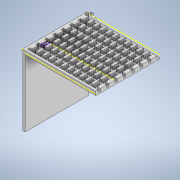
# Autodesk Inventor part: Garbage collectorBar
Saved by Autodesk Inventor 2022 (Build 260153000, 153)
## iProperties
Created: 2022-03-28
Part Number: Garbage collectorBar
Material: Generic
Document SubType Name: Modeling
Designer: Aditya Gupte
Density: 1 g/cm^3
Appearance: Default
Author: Aditya Gupte
Autodesk Inventor part; units mm, degrees
ref_plane "YZ Plane" through (0, 0, 0) normal (1, 0, 0) x (0, 1, 0)
ref_plane "XZ Plane" through (0, 0, 0) normal (0, 1, 0) x (-1, 0, 0)
ref_plane "XY Plane" through (0, 0, 0) normal (0, 0, 1) x (1, 0, 0)
sketch "Sketch1" plane through (0, 0, 0) normal (0, 0, 1) x (1, 0, 0)
  line L0 (0, 0) -> (15000, 0)
  line L1 (0, 0) -> (0, 14450)
  line L2 (0, 14450) -> (500, 14450)
  line L3 (500, 14450) -> (500, 300)
  line L4 (500, 300) -> (14950, 300)
  line L5 (14950, 300) -> (14950, 0)
  dimension "d0" = 15000
  dimension "d1" = 14450
  dimension "d2" = 500
  dimension "d3" = 14150
  dimension "d4" = 14450
  constraints: 12 end point, 3 perpendicular, 2 horizontal, 1 point on line, 1 vertical
  measures "d0" distance of L0.start L0.end
  measures "d1" distance of L0.start L1.end
  measures "d2" distance of L1.end L2.end
  measures "d3" distance of L2.end L3.end
  measures "d4" distance of L3.end L4.end
extrude "Extrusion1" add sketch "Sketch1" against normal blind 13000
sketch "Sketch2" plane through (500, 300, 0) normal (0, 1, 0) x (1, 0, 0)
  line L0 (14450, 0) -> (0, 0) projected
  line L1 (0, 0) -> (0, 13000) projected
  line L2 (-500, 0) -> (-500, 13000) projected
  dimension "d8" = 500
  measures "d8" distance between parallel lines of L1 L2
sketch "Sketch3" plane through (500, 300, 0) normal (0, 1, 0) x (1, 0, 0)
  line L0 (14450, 0) -> (14450, 13000) projected
  line L1 (14450, 0) -> (0, 0) projected
  line L2 (14450, 450) -> (0, 450)
  line L3 (14450, 950) -> (0, 950)
  line L4 (0, 0) -> (0, 13000) projected
  line L5 (0, 0) -> (0, 450)
  line L6 (14450, 0) -> (14450, 450)
  line L7 (0, 950) -> (14450, 950)
  line L8 (14450, 950) -> (14450, 2170)
  line L9 (14450, 2170) -> (0, 2170)
  line L10 (0, 2170) -> (0, 950)
  line L11 (0, 2670) -> (14450, 2670)
  line L12 (14450, 2670) -> (14450, 3890)
  line L13 (14450, 3890) -> (0, 3890)
  line L14 (0, 3890) -> (0, 2670)
  line L15 (0, 4390) -> (14450, 4390)
  line L16 (14450, 4390) -> (14450, 5610)
  line L17 (14450, 5610) -> (0, 5610)
  line L18 (0, 5610) -> (0, 4390)
  line L19 (0, 6110) -> (14450, 6110)
  line L20 (14450, 6110) -> (14450, 7330)
  line L21 (14450, 7330) -> (0, 7330)
  line L22 (0, 7330) -> (0, 6110)
  line L23 (0, 7830) -> (14450, 7830)
  line L24 (14450, 7830) -> (14450, 9050)
  line L25 (14450, 9050) -> (0, 9050)
  line L26 (0, 9050) -> (0, 7830)
  line L27 (0, 9550) -> (14450, 9550)
  line L28 (14450, 9550) -> (14450, 10770)
  line L29 (14450, 10770) -> (0, 10770)
  line L30 (0, 10770) -> (0, 9550)
  line L31 (0, 11270) -> (14450, 11270)
  line L32 (14450, 11270) -> (14450, 12490)
  line L33 (14450, 12490) -> (0, 12490)
  line L34 (0, 12490) -> (0, 11270)
  point P0 (-500, 0)
  point P1 (0, 5610)
  point P2 (0, 7330)
  point P3 (0, 10770)
  point P4 (0, 12490)
  dimension "d9" = 450
  dimension "d10" = 14450
  dimension "d11" = 14450
  dimension "d12" = 500
  dimension "d13" = 1220
  dimension "d14" = 500
  dimension "d15" = 1220
  dimension "d16" = 1220
  dimension "d17" = 500
  dimension "d18" = 1220
  dimension "d19" = 500
  dimension "d20" = 1220
  dimension "d21" = 500
  dimension "d22" = 1220
  dimension "d23" = 500
  dimension "d24" = 1220
  dimension "d25" = 500
  constraints: 64 end point, 14 parallel, 9 horizontal, 7 perpendicular, 1 vertical, 17 other
  measures "d9" distance from line of L2.start L1
  measures "d10" distance of L2.start L2.end
  measures "d11" distance of L3.start L3.end
  measures "d12" distance between parallel lines of L3 L2
  measures "d13" distance of L8.end L7.end
  measures "d14" distance between parallel lines of L11 L9
  measures "d15" distance of L11.end L12.end
  measures "d16" distance of L16.end L15.end
  measures "d17" distance between parallel lines of L15 L13
  measures "d18" distance of L20.end L19.end
  measures "d19" distance between parallel lines of L19 L17
  measures "d20" distance of L24.end L23.end
  measures "d21" distance between parallel lines of L23 L21
  measures "d22" distance of L28.end L27.end
  measures "d23" distance between parallel lines of L27 L25
  measures "d24" distance of L32.end L31.end
  measures "d25" distance between parallel lines of L31 L29
extrude "Extrusion2" add sketch "Sketch3" along normal blind 500 contours L3 L4 L9 L0 | L11 L4 L13 L0 | L15 L4 L17 L0 | L19 L4 L21 L0 | L23 L4 L25 L0 | L27 L4 L29 L0 | L31 L4 L33 L0
sketch "Sketch4" plane through (500, 300, 0) normal (0, 1, 0) x (1, 0, 0)
  line L0 (0, 0) -> (0, 13000) projected
  line L1 (14450, 0) -> (14450, 13000) projected
  line L2 (0, 0) -> (14450, 0)
  line L3 (14450, 0) -> (14450, 450)
  line L4 (14450, 450) -> (0, 450)
  line L5 (0, 450) -> (0, 0)
  point P0 (-500, 0)
  dimension "d28" = 450
  constraints: 8 end point, 2 parallel, 1 horizontal, 1 perpendicular, 1 point on line
  measures "d28" distance of L3.end L2.end
extrude "Extrusion3" add sketch "Sketch4" along normal blind 500
sketch "Sketch5" plane through (500, 800, 0) normal (0, 1, 0) x (1, 0, 0)
  line L0 (0, 12490) -> (14450, 12490) projected
  line L1 (0, 11270) -> (14450, 11270) projected
  line L2 (500, 12490) -> (1250, 12490)
  line L3 (1250, 12490) -> (1250, 11270)
  line L4 (1250, 11270) -> (500, 11270)
  line L5 (500, 11270) -> (500, 12490)
  line L6 (0, 0) -> (0, 13000) projected
  line L7 (1750, 12490) -> (2500, 12490)
  line L8 (2500, 12490) -> (2500, 11270)
  line L9 (2500, 11270) -> (1750, 11270)
  line L10 (1750, 11270) -> (1750, 12490)
  line L11 (3000, 12490) -> (3750, 12490)
  line L12 (3750, 12490) -> (3750, 11270)
  line L13 (3750, 11270) -> (3000, 11270)
  line L14 (3000, 11270) -> (3000, 12490)
  line L15 (4250, 12490) -> (5000, 12490)
  line L16 (5000, 12490) -> (5000, 11270)
  line L17 (5000, 11270) -> (4250, 11270)
  line L18 (4250, 11270) -> (4250, 12490)
  line L19 (5500, 12490) -> (6250, 12490)
  line L20 (6250, 12490) -> (6250, 11270)
  line L21 (6250, 11270) -> (5500, 11270)
  line L22 (5500, 11270) -> (5500, 12490)
  line L23 (6750, 12490) -> (7500, 12490)
  line L24 (7500, 12490) -> (7500, 11270)
  line L25 (7500, 11270) -> (6750, 11270)
  line L26 (6750, 11270) -> (6750, 12490)
  line L27 (8000, 12490) -> (8750, 12490)
  line L28 (8750, 12490) -> (8750, 11270)
  line L29 (8750, 11270) -> (8000, 11270)
  line L30 (8000, 11270) -> (8000, 12490)
  line L31 (9250, 12490) -> (10000, 12490)
  line L32 (10000, 12490) -> (10000, 11270)
  line L33 (10000, 11270) -> (9250, 11270)
  line L34 (9250, 11270) -> (9250, 12490)
  line L35 (10500, 12490) -> (11250, 12490)
  line L36 (11250, 12490) -> (11250, 11270)
  line L37 (11250, 11270) -> (10500, 11270)
  line L38 (10500, 11270) -> (10500, 12490)
  line L39 (11750, 12490) -> (12500, 12490)
  line L40 (12500, 12490) -> (12500, 11270)
  line L41 (12500, 11270) -> (11750, 11270)
  line L42 (11750, 11270) -> (11750, 12490)
  line L43 (13000, 12490) -> (13750, 12490)
  line L44 (13750, 12490) -> (13750, 11270)
  line L45 (13750, 11270) -> (13000, 11270)
  line L46 (13000, 11270) -> (13000, 12490)
  point P0 (-500, 0)
  point P1 (2500, 12490)
  point P2 (500, 11270)
  point P3 (1250, 12490)
  dimension "d31" = 750
  dimension "d32" = 500
  dimension "d33" = 750
  dimension "d34" = 500
  dimension "d35" = 750
  dimension "d36" = 500
  dimension "d37" = 750
  dimension "d38" = 500
  dimension "d39" = 750
  dimension "d40" = 500
  dimension "d41" = 750
  dimension "d42" = 500
  dimension "d43" = 750
  dimension "d44" = 500
  dimension "d45" = 750
  dimension "d46" = 500
  dimension "d47" = 750
  dimension "d48" = 500
  dimension "d49" = 750
  dimension "d50" = 500
  dimension "d51" = 750
  dimension "d52" = 500
  constraints: 88 end point, 22 parallel, 11 horizontal, 11 perpendicular, 24 other
  measures "d31" distance of L3.end L4.end
  measures "d32" distance between parallel lines of L5 L6
  measures "d33" distance of L8.end L9.end
  measures "d34" distance between parallel lines of L10 L3
  measures "d35" distance of L12.end L13.end
  measures "d36" distance between parallel lines of L14 L8
  measures "d37" distance of L16.end L17.end
  measures "d38" distance between parallel lines of L18 L12
  measures "d39" distance of L20.end L21.end
  measures "d40" distance between parallel lines of L22 L16
  measures "d41" distance of L24.end L25.end
  measures "d42" distance between parallel lines of L26 L20
  measures "d43" distance of L28.end L29.end
  measures "d44" distance between parallel lines of L30 L24
  measures "d45" distance of L32.end L33.end
  measures "d46" distance between parallel lines of L34 L28
  measures "d47" distance of L36.end L37.end
  measures "d48" distance between parallel lines of L38 L32
  measures "d49" distance of L40.end L41.end
  measures "d50" distance between parallel lines of L42 L36
  measures "d51" distance of L44.end L45.end
  measures "d52" distance between parallel lines of L46 L40
extrude "Extrusion4" cut sketch "Sketch5" against normal through all contours L0 L3 L1 L5 | L0 L8 L1 L10 | L0 L12 L1 L14 | L0 L16 L1 L18 | L0 L20 L1 L22 | L0 L24 L1 L26 | L0 L28 L1 L30 | L0 L32 L1 L34 | L0 L36 L1 L38 | L0 L40 L1 L42 | L0 L44 L1 L46
sketch "Sketch6" plane through (500, 800, 0) normal (0, 1, 0) x (1, 0, 0)
  line L0 (14450, 10770) -> (0, 10770) projected
  line L1 (14450, 9550) -> (0, 9550) projected
  line L2 (500, 10770) -> (1250, 10770)
  line L3 (1250, 10770) -> (1250, 9550)
  line L4 (1250, 9550) -> (500, 9550)
  line L5 (500, 9550) -> (500, 10770)
  line L6 (0, 0) -> (0, 13000) projected
  line L7 (1750, 10770) -> (2500, 10770)
  line L8 (2500, 10770) -> (2500, 9550)
  line L9 (2500, 9550) -> (1750, 9550)
  line L10 (1750, 9550) -> (1750, 10770)
  line L11 (3000, 10770) -> (3750, 10770)
  line L12 (3750, 10770) -> (3750, 9550)
  line L13 (3750, 9550) -> (3000, 9550)
  line L14 (3000, 9550) -> (3000, 10770)
  line L15 (4250, 10770) -> (5000, 10770)
  line L16 (5000, 10770) -> (5000, 9550)
  line L17 (5000, 9550) -> (4250, 9550)
  line L18 (4250, 9550) -> (4250, 10770)
  line L19 (5500, 10770) -> (6250, 10770)
  line L20 (6250, 10770) -> (6250, 9550)
  line L21 (6250, 9550) -> (5500, 9550)
  line L22 (5500, 9550) -> (5500, 10770)
  line L23 (6750, 10770) -> (7500, 10770)
  line L24 (7500, 10770) -> (7500, 9550)
  line L25 (7500, 9550) -> (6750, 9550)
  line L26 (6750, 9550) -> (6750, 10770)
  line L27 (8000, 10770) -> (8750, 10770)
  line L28 (8750, 10770) -> (8750, 9550)
  line L29 (8750, 9550) -> (8000, 9550)
  line L30 (8000, 9550) -> (8000, 10770)
  line L31 (9250, 10770) -> (10000, 10770)
  line L32 (10000, 10770) -> (10000, 9550)
  line L33 (10000, 9550) -> (9250, 9550)
  line L34 (9250, 9550) -> (9250, 10770)
  line L35 (10500, 10770) -> (11250, 10770)
  line L36 (11250, 10770) -> (11250, 9550)
  line L37 (11250, 9550) -> (10500, 9550)
  line L38 (10500, 9550) -> (10500, 10770)
  line L39 (11750, 10770) -> (12500, 10770)
  line L40 (12500, 10770) -> (12500, 9550)
  line L41 (12500, 9550) -> (11750, 9550)
  line L42 (11750, 9550) -> (11750, 10770)
  line L43 (13000, 10770) -> (13750, 10770)
  line L44 (13750, 10770) -> (13750, 9550)
  line L45 (13750, 9550) -> (13000, 9550)
  line L46 (13000, 9550) -> (13000, 10770)
  line L47 (0, 9050) -> (14450, 9050) projected
  line L48 (500, 9050) -> (1250, 9050)
  line L49 (1250, 9050) -> (1250, 7803.8278)
  line L50 (1250, 7803.8278) -> (500, 7803.8278)
  line L51 (500, 7803.8278) -> (500, 9050)
  line L52 (1750, 9050) -> (2500, 9050)
  line L53 (2500, 9050) -> (2500, 7803.8278)
  line L54 (2500, 7803.8278) -> (1750, 7803.8278)
  line L55 (1750, 7803.8278) -> (1750, 9050)
  line L56 (3000, 9050) -> (3750, 9050)
  line L57 (3750, 9050) -> (3750, 7803.8278)
  line L58 (3750, 7803.8278) -> (3000, 7803.8278)
  line L59 (3000, 7803.8278) -> (3000, 9050)
  line L60 (4250, 9050) -> (5000, 9050)
  line L61 (5000, 9050) -> (5000, 7803.8278)
  line L62 (5000, 7803.8278) -> (4250, 7803.8278)
  line L63 (4250, 7803.8278) -> (4250, 9050)
  line L64 (5500, 9050) -> (6250, 9050)
  line L65 (6250, 9050) -> (6250, 7803.8278)
  line L66 (6250, 7803.8278) -> (5500, 7803.8278)
  line L67 (5500, 7803.8278) -> (5500, 9050)
  line L68 (6750, 9050) -> (7500, 9050)
  line L69 (7500, 9050) -> (7500, 7803.8278)
  line L70 (7500, 7803.8278) -> (6750, 7803.8278)
  line L71 (6750, 7803.8278) -> (6750, 9050)
  line L72 (8000, 9050) -> (8750, 9050)
  line L73 (8750, 9050) -> (8750, 7803.8278)
  line L74 (8750, 7803.8278) -> (8000, 7803.8278)
  line L75 (8000, 7803.8278) -> (8000, 9050)
  line L76 (0, 7830) -> (14450, 7830) projected
  line L77 (9250, 9050) -> (10000, 9050)
  line L78 (10000, 9050) -> (10000, 7830)
  line L79 (10000, 7830) -> (9250, 7830)
  line L80 (9250, 7830) -> (9250, 9050)
  line L81 (10500, 9050) -> (11250, 9050)
  line L82 (11250, 9050) -> (11250, 7830)
  line L83 (11250, 7830) -> (10500, 7830)
  line L84 (10500, 7830) -> (10500, 9050)
  line L85 (11750, 9050) -> (12500, 9050)
  line L86 (12500, 9050) -> (12500, 7830)
  line L87 (12500, 7830) -> (11750, 7830)
  line L88 (11750, 7830) -> (11750, 9050)
  line L89 (13000, 9050) -> (13750, 9050)
  line L90 (13750, 9050) -> (13750, 7830)
  line L91 (13750, 7830) -> (13000, 7830)
  line L92 (13000, 7830) -> (13000, 9050)
  line L93 (14450, 6110) -> (0, 6110) projected
  line L94 (500, 7312.9157) -> (1250, 7312.9157)
  line L95 (1250, 7312.9157) -> (1250, 6110)
  line L96 (1250, 6110) -> (500, 6110)
  line L97 (500, 6110) -> (500, 7312.9157)
  line L98 (1750, 7312.9157) -> (2500, 7312.9157)
  line L99 (2500, 7312.9157) -> (2500, 6110)
  line L100 (2500, 6110) -> (1750, 6110)
  line L101 (1750, 6110) -> (1750, 7312.9157)
  line L102 (3000, 7312.9157) -> (3750, 7312.9157)
  line L103 (3750, 7312.9157) -> (3750, 6110)
  line L104 (3750, 6110) -> (3000, 6110)
  line L105 (3000, 6110) -> (3000, 7312.9157)
  line L106 (4250, 7312.9157) -> (5000, 7312.9157)
  line L107 (5000, 7312.9157) -> (5000, 6110)
  line L108 (5000, 6110) -> (4250, 6110)
  line L109 (4250, 6110) -> (4250, 7312.9157)
  line L110 (0, 7330) -> (14450, 7330) projected
  line L111 (5500, 7330) -> (6250, 7330)
  line L112 (6250, 7330) -> (6250, 6110)
  line L113 (6250, 6110) -> (5500, 6110)
  line L114 (5500, 6110) -> (5500, 7330)
  line L115 (6750, 7330) -> (7500, 7330)
  line L116 (7500, 7330) -> (7500, 6110)
  line L117 (7500, 6110) -> (6750, 6110)
  line L118 (6750, 6110) -> (6750, 7330)
  line L119 (8000, 7330) -> (8750, 7330)
  line L120 (8750, 7330) -> (8750, 6110)
  line L121 (8750, 6110) -> (8000, 6110)
  line L122 (8000, 6110) -> (8000, 7330)
  line L123 (9250, 7330) -> (10000, 7330)
  line L124 (10000, 7330) -> (10000, 6110)
  line L125 (10000, 6110) -> (9250, 6110)
  line L126 (9250, 6110) -> (9250, 7330)
  line L127 (10500, 7330) -> (11250, 7330)
  line L128 (11250, 7330) -> (11250, 6110)
  line L129 (11250, 6110) -> (10500, 6110)
  line L130 (10500, 6110) -> (10500, 7330)
  line L131 (11750, 7330) -> (12500, 7330)
  line L132 (12500, 7330) -> (12500, 6110)
  line L133 (12500, 6110) -> (11750, 6110)
  line L134 (11750, 6110) -> (11750, 7330)
  line L135 (13000, 7312.9157) -> (13750, 7312.9157)
  line L136 (13750, 7312.9157) -> (13750, 6110)
  line L137 (13750, 6110) -> (13000, 6110)
  line L138 (13000, 6110) -> (13000, 7312.9157)
  line L139 (14450, 4390) -> (0, 4390) projected
  line L140 (500, 5594.7232) -> (1250, 5594.7232)
  line L141 (1250, 5594.7232) -> (1250, 4390)
  line L142 (1250, 4390) -> (500, 4390)
  line L143 (500, 4390) -> (500, 5594.7232)
  line L144 (1750, 5594.7232) -> (2500, 5594.7232)
  line L145 (2500, 5594.7232) -> (2500, 4390)
  line L146 (2500, 4390) -> (1750, 4390)
  line L147 (1750, 4390) -> (1750, 5594.7232)
  line L148 (3000, 5594.7232) -> (3750, 5594.7232)
  line L149 (3750, 5594.7232) -> (3750, 4390)
  line L150 (3750, 4390) -> (3000, 4390)
  line L151 (3000, 4390) -> (3000, 5594.7232)
  line L152 (4250, 5594.7232) -> (5000, 5594.7232)
  line L153 (5000, 5594.7232) -> (5000, 4390)
  line L154 (5000, 4390) -> (4250, 4390)
  line L155 (4250, 4390) -> (4250, 5594.7232)
  line L156 (5500, 5594.7232) -> (6250, 5594.7232)
  line L157 (6250, 5594.7232) -> (6250, 4390)
  line L158 (6250, 4390) -> (5500, 4390)
  line L159 (5500, 4390) -> (5500, 5594.7232)
  line L160 (0, 5610) -> (14450, 5610) projected
  line L161 (6750, 5610) -> (7500, 5610)
  line L162 (7500, 5610) -> (7500, 4390)
  line L163 (7500, 4390) -> (6750, 4390)
  line L164 (6750, 4390) -> (6750, 5610)
  line L165 (8000, 5610) -> (8750, 5610)
  line L166 (8750, 5610) -> (8750, 4390)
  line L167 (8750, 4390) -> (8000, 4390)
  line L168 (8000, 4390) -> (8000, 5610)
  line L169 (9250, 5610) -> (10000, 5610)
  line L170 (10000, 5610) -> (10000, 4390)
  line L171 (10000, 4390) -> (9250, 4390)
  line L172 (9250, 4390) -> (9250, 5610)
  line L173 (10500, 5610) -> (11250, 5610)
  line L174 (11250, 5610) -> (11250, 4390)
  line L175 (11250, 4390) -> (10500, 4390)
  line L176 (10500, 4390) -> (10500, 5610)
  line L177 (11750, 5610) -> (12500, 5610)
  line L178 (12500, 5610) -> (12500, 4390)
  line L179 (12500, 4390) -> (11750, 4390)
  line L180 (11750, 4390) -> (11750, 5610)
  line L181 (13000, 5610) -> (13750, 5610)
  line L182 (13750, 5610) -> (13750, 4390)
  line L183 (13750, 4390) -> (13000, 4390)
  line L184 (13000, 4390) -> (13000, 5610)
  line L185 (0, 3890) -> (14450, 3890) projected
  line L186 (0, 2670) -> (14450, 2670) projected
  line L187 (500, 3890) -> (1250, 3890)
  line L188 (1250, 3890) -> (1250, 2670)
  line L189 (1250, 2670) -> (500, 2670)
  line L190 (500, 2670) -> (500, 3890)
  line L191 (1750, 3890) -> (2500, 3890)
  line L192 (2500, 3890) -> (2500, 2670)
  line L193 (2500, 2670) -> (1750, 2670)
  line L194 (1750, 2670) -> (1750, 3890)
  line L195 (3000, 3890) -> (3750, 3890)
  line L196 (3750, 3890) -> (3750, 2670)
  line L197 (3750, 2670) -> (3000, 2670)
  line L198 (3000, 2670) -> (3000, 3890)
  line L199 (4250, 3890) -> (5000, 3890)
  line L200 (5000, 3890) -> (5000, 2670)
  line L201 (5000, 2670) -> (4250, 2670)
  line L202 (4250, 2670) -> (4250, 3890)
  line L203 (5500, 3890) -> (6250, 3890)
  line L204 (6250, 3890) -> (6250, 2670)
  line L205 (6250, 2670) -> (5500, 2670)
  line L206 (5500, 2670) -> (5500, 3890)
  line L207 (6750, 3890) -> (7500, 3890)
  line L208 (7500, 3890) -> (7500, 2670)
  line L209 (7500, 2670) -> (6750, 2670)
  line L210 (6750, 2670) -> (6750, 3890)
  line L211 (8000, 3890) -> (8750, 3890)
  line L212 (8750, 3890) -> (8750, 2670)
  line L213 (8750, 2670) -> (8000, 2670)
  line L214 (8000, 2670) -> (8000, 3890)
  line L215 (9250, 3890) -> (10000, 3890)
  line L216 (10000, 3890) -> (10000, 2670)
  line L217 (10000, 2670) -> (9250, 2670)
  line L218 (9250, 2670) -> (9250, 3890)
  line L219 (10500, 3890) -> (11250, 3890)
  line L220 (11250, 3890) -> (11250, 2670)
  line L221 (11250, 2670) -> (10500, 2670)
  line L222 (10500, 2670) -> (10500, 3890)
  line L223 (11750, 3890) -> (12500, 3890)
  line L224 (12500, 3890) -> (12500, 2670)
  line L225 (12500, 2670) -> (11750, 2670)
  line L226 (11750, 2670) -> (11750, 3890)
  line L227 (13000, 3890) -> (13750, 3890)
  line L228 (13750, 3890) -> (13750, 2670)
  line L229 (13750, 2670) -> (13000, 2670)
  line L230 (13000, 2670) -> (13000, 3890)
  line L231 (14450, 2170) -> (0, 2170) projected
  line L232 (0, 950) -> (14450, 950) projected
  line L233 (500, 2170) -> (1250, 2170)
  line L234 (1250, 2170) -> (1250, 950)
  line L235 (1250, 950) -> (500, 950)
  line L236 (500, 950) -> (500, 2170)
  line L237 (1750, 2170) -> (2500, 2170)
  line L238 (2500, 2170) -> (2500, 950)
  line L239 (2500, 950) -> (1750, 950)
  line L240 (1750, 950) -> (1750, 2170)
  line L241 (3000, 2170) -> (3750, 2170)
  line L242 (3750, 2170) -> (3750, 950)
  line L243 (3750, 950) -> (3000, 950)
  line L244 (3000, 950) -> (3000, 2170)
  line L245 (4250, 2170) -> (5000, 2170)
  line L246 (5000, 2170) -> (5000, 950)
  line L247 (5000, 950) -> (4250, 950)
  line L248 (4250, 950) -> (4250, 2170)
  line L249 (5500, 2170) -> (6250, 2170)
  line L250 (6250, 2170) -> (6250, 950)
  line L251 (6250, 950) -> (5500, 950)
  line L252 (5500, 950) -> (5500, 2170)
  line L253 (6750, 2170) -> (7500, 2170)
  line L254 (7500, 2170) -> (7500, 950)
  line L255 (7500, 950) -> (6750, 950)
  line L256 (6750, 950) -> (6750, 2170)
  line L257 (8000, 2170) -> (8750, 2170)
  line L258 (8750, 2170) -> (8750, 950)
  line L259 (8750, 950) -> (8000, 950)
  line L260 (8000, 950) -> (8000, 2170)
  line L261 (9250, 2170) -> (10000, 2170)
  line L262 (10000, 2170) -> (10000, 950)
  line L263 (10000, 950) -> (9250, 950)
  line L264 (9250, 950) -> (9250, 2170)
  line L265 (10500, 2170) -> (11250, 2170)
  line L266 (11250, 2170) -> (11250, 950)
  line L267 (11250, 950) -> (10500, 950)
  line L268 (10500, 950) -> (10500, 2170)
  line L269 (11750, 2170) -> (12500, 2170)
  line L270 (12500, 2170) -> (12500, 950)
  line L271 (12500, 950) -> (11750, 950)
  line L272 (11750, 950) -> (11750, 2170)
  line L273 (13000, 2170) -> (13750, 2170)
  line L274 (13750, 2170) -> (13750, 950)
  line L275 (13750, 950) -> (13000, 950)
  line L276 (13000, 950) -> (13000, 2170)
  point P0 (-500, 0)
  point P1 (10000, 10770)
  point P2 (2500, 10770)
  point P3 (500, 9550)
  point P4 (1250, 10770)
  point P5 (1250, 9050)
  point P6 (9250, 7830)
  point P7 (10000, 9050)
  dimension "d55" = 750
  dimension "d56" = 500
  dimension "d57" = 750
  dimension "d58" = 500
  dimension "d59" = 750
  dimension "d60" = 500
  dimension "d61" = 750
  dimension "d62" = 500
  dimension "d63" = 750
  dimension "d64" = 500
  dimension "d65" = 750
  dimension "d66" = 500
  dimension "d67" = 750
  dimension "d68" = 500
  dimension "d69" = 750
  dimension "d70" = 500
  dimension "d71" = 750
  dimension "d72" = 500
  dimension "d73" = 750
  dimension "d74" = 500
  dimension "d75" = 750
  dimension "d76" = 500
  dimension "d77" = 500
  dimension "d78" = 500
  constraints: 528 end point, 132 parallel, 66 horizontal, 66 perpendicular, 58 point on line, 76 other
  measures "d55" distance of L3.end L4.end
  measures "d56" distance of the line from the sketch origin of L5
  measures "d57" distance of L8.end L9.end
  measures "d58" distance between parallel lines of L10 L3
  measures "d59" distance of L12.end L13.end
  measures "d60" distance between parallel lines of L14 L8
  measures "d61" distance of L16.end L17.end
  measures "d62" distance between parallel lines of L18 L12
  measures "d63" distance of L20.end L21.end
  measures "d64" distance between parallel lines of L22 L16
  measures "d65" distance of L24.end L25.end
  measures "d66" distance between parallel lines of L26 L20
  measures "d67" distance of L28.end L29.end
  measures "d68" distance between parallel lines of L30 L24
  measures "d69" distance of L32.end L33.end
  measures "d70" distance between parallel lines of L34 L28
  measures "d71" distance of L36.end L37.end
  measures "d72" distance between parallel lines of L38 L32
  measures "d73" distance of L40.end L41.end
  measures "d74" distance between parallel lines of L42 L36
  measures "d75" distance of L44.end L45.end
  measures "d76" distance between parallel lines of L46 L40
  measures "d77" distance of the line from the sketch origin of L51
  measures "d78" distance between parallel lines of L55 L49
extrude "Extrusion5" cut sketch "Sketch6" against normal through all contours L44 L1 L46 L0 | L40 L1 L42 L0 | L36 L1 L38 L0 | L32 L1 L34 L0 | L28 L1 L30 L0 | L24 L1 L26 L0 | L20 L1 L22 L0 | L16 L1 L18 L0 | L12 L1 L14 L0 | L8 L1 L10 L0 | L3 L1 L5 L0 | L84 L47 L82 L76 | L88 L47 L86 L76 | L92 L47 L90 L76
extrude "Extrusion6" cut sketch "Sketch6" against normal through all contours L143 L140 L141 L139 | L160 L162 L139 L164 | L147 L144 L145 L139 | L160 L166 L139 L168 | L139 L159 L156 L157 | L151 L148 L149 L139 | L160 L170 L139 L172 | L139 L155 L152 L153 | L160 L174 L139 L176 | L160 L178 L139 L180 | L160 L182 L139 L184 | L97 L94 L95 L93 | L110 L112 L93 L114 | L101 L98 L99 L93 | L110 L116 L93 L118 | L93 L109 L106 L107 | L105 L102 L103 L93 | L110 L120 L93 L122 | L110 L124 L93 L126 | L110 L128 L93 L130 | L110 L132 L93 L134 | L76 L49 L50 L51 | L51 L47 L49 L76 | L76 L53 L54 L55 | L55 L47 L53 L76 | L76 L57 L58 L59 | L59 L47 L57 L76 | L76 L61 L62 L63 | L63 L47 L61 L76 | L76 L65 L66 L67 | L67 L47 L65 L76 | L76 L69 L70 L71 | L71 L47 L69 L76 | L76 L73 L74 L75 | L75 L47 L73 L76 | L80 L47 L78 L76 | L93 L138 L135 L136
sketch "Sketch7" plane through (500, 800, 0) normal (0, 1, 0) x (1, 0, 0)
  line L0 (0, 3890) -> (14450, 3890) projected
  line L1 (487.0993, 3890) -> (1237.0993, 3890)
  line L2 (1237.0993, 3890) -> (1237.0993, 2624.641)
  line L3 (1237.0993, 2624.641) -> (487.0993, 2624.641)
  line L4 (487.0993, 2624.641) -> (487.0993, 3890)
  point P0 (-500, 0)
  dimension "d83" = 750
  constraints: 8 end point, 2 parallel, 1 horizontal, 1 perpendicular, 1 point on line
  measures "d83" distance of L2.end L3.end
extrude "Extrusion7" cut sketch "Sketch7" against normal blind 10
extrude "Extrusion8" cut sketch "Sketch7" against normal up to next
sketch "Sketch8" plane through (500, 800, 0) normal (0, 1, 0) x (1, 0, 0)
  line L0 (1237.0993, 3890) -> (14450, 3890) projected
  line L1 (14450, 2670) -> (1237.0993, 2670) projected
  line L2 (1760.2519, 3890) -> (2510.2519, 3890)
  line L3 (2510.2519, 3890) -> (2510.2519, 2670)
  line L4 (2510.2519, 2670) -> (1760.2519, 2670)
  line L5 (1760.2519, 2670) -> (1760.2519, 3890)
  line L6 (3010.4779, 3890) -> (3775.0706, 3890)
  line L7 (3775.0706, 3890) -> (3775.0706, 2670)
  line L8 (3775.0706, 2670) -> (3010.4779, 2670)
  line L9 (3010.4779, 2670) -> (3010.4779, 3890)
  line L10 (4246.4306, 3890) -> (4996.4306, 3890)
  line L11 (4996.4306, 3890) -> (4996.4306, 2670)
  line L12 (4996.4306, 2670) -> (4246.4306, 2670)
  line L13 (4246.4306, 2670) -> (4246.4306, 3890)
  point P0 (-500, 0)
  dimension "d88" = 750
  dimension "d89" = 750
  constraints: 24 end point, 6 parallel, 6 point on line, 3 horizontal, 3 perpendicular
  measures "d88" distance of L3.end L4.end
  measures "d89" distance of L11.end L12.end
extrude "Extrusion9" cut sketch "Sketch8" against normal up to next contours L0 L3 L1 L5 | L0 L7 L1 L9 | L0 L11 L1 L13
sketch "Sketch9" plane through (500, 800, 0) normal (0, 1, 0) x (1, 0, 0)
  line L0 (14450, 3890) -> (4996.4306, 3890) projected
  line L1 (14450, 2670) -> (4996.4306, 2670) projected
  line L2 (5506.9149, 3890) -> (6256.9149, 3890)
  line L3 (6256.9149, 3890) -> (6256.9149, 2670)
  line L4 (6256.9149, 2670) -> (5506.9149, 2670)
  line L5 (5506.9149, 2670) -> (5506.9149, 3890)
  line L6 (6756.9149, 3890) -> (7521.4013, 3890)
  line L7 (7521.4013, 3890) -> (7521.4013, 2670)
  line L8 (7521.4013, 2670) -> (6756.9149, 2670)
  line L9 (6756.9149, 2670) -> (6756.9149, 3890)
  line L10 (8021.4013, 3890) -> (8785.1443, 3890)
  line L11 (8785.1443, 3890) -> (8785.1443, 2670)
  line L12 (8785.1443, 2670) -> (8021.4013, 2670)
  line L13 (8021.4013, 2670) -> (8021.4013, 3890)
  line L14 (9285.1443, 3890) -> (10054.0905, 3890)
  line L15 (10054.0905, 3890) -> (10054.0905, 2670)
  line L16 (10054.0905, 2670) -> (9285.1443, 2670)
  line L17 (9285.1443, 2670) -> (9285.1443, 3890)
  line L18 (4250, 4390) -> (4250, 5594.7232) projected
  line L19 (3750, 5594.7232) -> (3750, 4390) projected
  line L20 (10554.0905, 3890) -> (11220.6318, 3890)
  line L21 (11220.6318, 3890) -> (11220.6318, 2670)
  line L22 (11220.6318, 2670) -> (10554.0905, 2670)
  line L23 (10554.0905, 2670) -> (10554.0905, 3890)
  line L24 (11720.6318, 3890) -> (12507.9159, 3890)
  line L25 (12507.9159, 3890) -> (12507.9159, 2670)
  line L26 (12507.9159, 2670) -> (11720.6318, 2670)
  line L27 (11720.6318, 2670) -> (11720.6318, 3890)
  line L28 (13007.9159, 3890) -> (13750, 3890)
  line L29 (13750, 3890) -> (13750, 2670)
  line L30 (13750, 2670) -> (13007.9159, 2670)
  line L31 (13007.9159, 2670) -> (13007.9159, 3890)
  line L32 (14450, 2670) -> (14450, 3890) projected
  point P0 (-500, 0)
  dimension "d92" = 750
  dimension "d93" = 750
  dimension "d94" = 500
  dimension "d95" = 500
  dimension "d96" = 500
  dimension "d97" = 500
  dimension "d98" = 500
  dimension "d99" = 500
  dimension "d100" = 500
  dimension "d101" = 700
  constraints: 56 end point, 14 parallel, 14 point on line, 7 horizontal, 7 perpendicular
  measures "d92" distance of L3.end L4.end
  measures "d93" distance between parallel lines of L3 L5
  measures "d94" distance between parallel lines of L18 L19
  measures "d95" distance between parallel lines of L9 L3
  measures "d96" distance between parallel lines of L13 L7
  measures "d97" distance between parallel lines of L17 L11
  measures "d98" distance between parallel lines of L23 L15
  measures "d99" distance between parallel lines of L27 L21
  measures "d100" distance between parallel lines of L31 L25
  measures "d101" distance between parallel lines of L32 L29
extrude "Extrusion10" cut sketch "Sketch9" against normal up to next contours L29 L1 L31 L0 | L25 L1 L27 L0 | L21 L1 L23 L0 | L15 L1 L17 L0 | L11 L1 L13 L0 | L7 L1 L9 L0 | L3 L1 L5 L0
sketch "Sketch10" plane through (500, 800, 0) normal (0, 1, 0) x (1, 0, 0)
  line L0 (14450, 2170) -> (0, 2170) projected
  line L1 (0, 950) -> (14450, 950) projected
  line L2 (480.0434, 2170) -> (1230.0434, 2170)
  line L3 (1230.0434, 2170) -> (1230.0434, 950)
  line L4 (1230.0434, 950) -> (480.0434, 950)
  line L5 (480.0434, 950) -> (480.0434, 2170)
  line L6 (1730.0434, 2170) -> (2480.0434, 2170)
  line L7 (2480.0434, 2170) -> (2480.0434, 950)
  line L8 (2480.0434, 950) -> (1730.0434, 950)
  line L9 (1730.0434, 950) -> (1730.0434, 2170)
  line L10 (2980.0434, 2170) -> (3730.0434, 2170)
  line L11 (3730.0434, 2170) -> (3730.0434, 950)
  line L12 (3730.0434, 950) -> (2980.0434, 950)
  line L13 (2980.0434, 950) -> (2980.0434, 2170)
  line L14 (4230.0434, 2170) -> (4980.0434, 2170)
  line L15 (4980.0434, 2170) -> (4980.0434, 950)
  line L16 (4980.0434, 950) -> (4230.0434, 950)
  line L17 (4230.0434, 950) -> (4230.0434, 2170)
  line L18 (5480.0434, 2170) -> (6230.0434, 2170)
  line L19 (6230.0434, 2170) -> (6230.0434, 950)
  line L20 (6230.0434, 950) -> (5480.0434, 950)
  line L21 (5480.0434, 950) -> (5480.0434, 2170)
  line L22 (6730.0434, 2170) -> (7480.0434, 2170)
  line L23 (7480.0434, 2170) -> (7480.0434, 950)
  line L24 (7480.0434, 950) -> (6730.0434, 950)
  line L25 (6730.0434, 950) -> (6730.0434, 2170)
  line L26 (7980.0434, 2170) -> (8730.0434, 2170)
  line L27 (8730.0434, 2170) -> (8730.0434, 950)
  line L28 (8730.0434, 950) -> (7980.0434, 950)
  line L29 (7980.0434, 950) -> (7980.0434, 2170)
  line L30 (9230.0434, 2170) -> (9980.0434, 2170)
  line L31 (9980.0434, 2170) -> (9980.0434, 950)
  line L32 (9980.0434, 950) -> (9230.0434, 950)
  line L33 (9230.0434, 950) -> (9230.0434, 2170)
  line L34 (10480.0434, 2170) -> (11230.0434, 2170)
  line L35 (11230.0434, 2170) -> (11230.0434, 950)
  line L36 (11230.0434, 950) -> (10480.0434, 950)
  line L37 (10480.0434, 950) -> (10480.0434, 2170)
  line L38 (11730.0434, 2170) -> (12480.0434, 2170)
  line L39 (12480.0434, 2170) -> (12480.0434, 950)
  line L40 (12480.0434, 950) -> (11730.0434, 950)
  line L41 (11730.0434, 950) -> (11730.0434, 2170)
  line L42 (12980.0434, 2170) -> (13750, 2170)
  line L43 (13750, 2170) -> (13750, 950)
  line L44 (13750, 950) -> (12980.0434, 950)
  line L45 (12980.0434, 950) -> (12980.0434, 2170)
  line L46 (14450, 950) -> (14450, 2170) projected
  point P0 (-500, 0)
  point P1 (480.0434, 950)
  dimension "d104" = 500
  dimension "d105" = 500
  dimension "d106" = 500
  dimension "d107" = 500
  dimension "d108" = 500
  dimension "d109" = 500
  dimension "d110" = 500
  dimension "d111" = 500
  dimension "d112" = 500
  dimension "d113" = 500
  dimension "d114" = 700
  dimension "d115" = 750
  dimension "d116" = 750
  dimension "d117" = 750
  dimension "d118" = 750
  dimension "d119" = 750
  dimension "d120" = 750
  dimension "d121" = 750
  dimension "d122" = 750
  dimension "d123" = 750
  dimension "d124" = 750
  dimension "d125" = 1220
  constraints: 88 end point, 22 parallel, 13 point on line, 11 horizontal, 11 perpendicular, 10 other
  measures "d104" distance between parallel lines of L9 L3
  measures "d105" distance between parallel lines of L17 L11
  measures "d106" distance between parallel lines of L13 L7
  measures "d107" distance between parallel lines of L21 L15
  measures "d108" distance between parallel lines of L25 L19
  measures "d109" distance between parallel lines of L29 L23
  measures "d110" distance between parallel lines of L33 L27
  measures "d111" distance between parallel lines of L37 L31
  measures "d112" distance between parallel lines of L41 L35
  measures "d113" distance between parallel lines of L45 L39
  measures "d114" distance between parallel lines of L46 L43
  measures "d115" distance between parallel lines of L3 L5
  measures "d116" distance between parallel lines of L7 L9
  measures "d117" distance between parallel lines of L11 L13
  measures "d118" distance between parallel lines of L15 L17
  measures "d119" distance between parallel lines of L19 L21
  measures "d120" distance between parallel lines of L23 L25
  measures "d121" distance between parallel lines of L27 L29
  measures "d122" distance between parallel lines of L31 L33
  measures "d123" distance between parallel lines of L35 L37
  measures "d124" distance between parallel lines of L39 L41
extrude "Extrusion11" cut sketch "Sketch10" against normal up to next contours L43 L1 L45 L0 | L39 L1 L41 L0 | L35 L1 L37 L0 | L31 L1 L33 L0 | L27 L1 L29 L0 | L23 L1 L25 L0 | L19 L1 L21 L0 | L15 L1 L17 L0 | L11 L1 L13 L0 | L7 L1 L9 L0 | L3 L1 L5 L0
sketch "Sketch11" plane through (0, 14450, 0) normal (0, 1, 0) x (1, 0, 0)
  line L0 (500, 0) -> (14950, 0) projected
  line L1 (0, 0) -> (0, 13000) projected
  line L2 (500, 0) -> (0, 0)
  line L3 (0, 0) -> (0, 13000)
  line L4 (0, 13000) -> (500, 13000)
  line L5 (500, 13000) -> (500, 0)
  constraints: 8 end point, 2 parallel, 1 horizontal, 1 perpendicular
extrude "Extrusion12" cut sketch "Sketch11" against normal up to surface (13650 mm away)
sketch "Sketch12" plane through (0, 0, 0) normal (0, -1, 0) x (1, 0, 0)
  line L0 (14950, -13000) -> (0, -13000) projected
  line L1 (0, -13000) -> (500, -13000)
  line L2 (500, -13000) -> (500, 0)
  line L3 (500, 0) -> (0, 0)
  line L4 (0, 0) -> (0, -13000)
  constraints: 8 end point, 2 parallel, 1 horizontal, 1 perpendicular
sketch "Sketch13" plane through (0, 0, -13000) normal (0, 0, -1) x (-1, 0, 0)
  line L0 (-14950, 800) -> (0, 800) projected
  point P0 (0, 0)
extrude "Extrusion13" add sketch "Sketch12" along normal blind 13650
body "Solid1"
